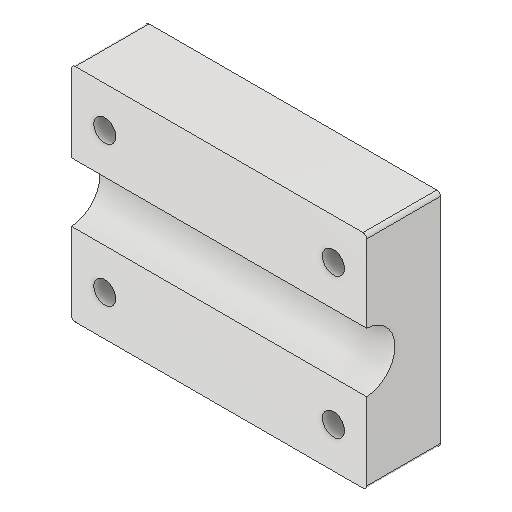
# Autodesk Inventor part: 3DP_PLA_Y_axis_linear_shaft_mount_clamp_with_endstop
Saved by Autodesk Inventor 2025 (Build 290162010, 162A)
## iProperties
Created: 2018-06-17
Part Number: 3DP_PLA_Y_axis_linear_shaft_mount_clamp_with_endstop
Material: ABS Plastic
Document SubType Name: Modeling
Designer: Andrzej
Density: 1.06 g/cm^3
Appearance: Smooth - White
Author: Andrzej
Autodesk Inventor part; units mm, degrees
ref_plane "YZ Plane" through (0, 0, 0) normal (1, 0, 0) x (0, 1, 0)
ref_plane "XZ Plane" through (0, 0, 0) normal (0, 1, 0) x (-1, 0, 0)
ref_plane "XY Plane" through (0, 0, 0) normal (0, 0, 1) x (1, 0, 0)
sketch "Sketch1" plane through (0, 0, 0) normal (0, 0, 1) x (1, 0, 0)
  line L0 (-26.9235, 18.928) -> (13.0765, 18.928)
  line L1 (13.0765, 18.928) -> (13.0765, -11.072)
  line L2 (13.0765, -11.072) -> (-26.9235, -11.072)
  line L3 (-26.9235, -11.072) -> (-26.9235, 18.928)
  point P0 (0, 0)
  dimension "d1" = 30
  dimension "d47" = 40
  constraints: 8 end point, 2 parallel, 1 horizontal, 1 perpendicular
  measures "d1" distance of L0.end L1.end
  measures "d47" distance of L1.end L2.end
extrude "Extrusion1" add sketch "Sketch1" along normal blind 10
sketch "Sketch2" plane through (13.0765, -11.072, 10) normal (1, 0, 0) x (0, 0, -1)
  line L0 (10, 30) -> (0, 30) projected
  line L1 (0, 0) -> (0, 30) projected
  line L2 (10, 0) -> (0, 0) projected
  circle A0 centre (-0.2, 15) radius 4.025
  line L3 (10, 30) -> (10, 0) projected
  dimension "d20" = 30
  dimension "d21" = 15
  dimension "d22" = 0.2
  dimension "d23" = 8.05
  constraints: 1 centre point, 1 coincident
  measures "d20" distance between parallel lines of L0 L2
  measures "d21" distance from line of L2 point (-0.2, 15)
  measures "d22" distance from line of L1 point (-0.2, 15)
  measures "d23" diameter of A0
extrude "Extrusion3" cut sketch "Sketch2" against normal through all contours A0 L1 | L1 A0
sketch "Sketch3" plane through (0, 0, 10) normal (0, 0, 1) x (1, 0, 0)
  line L0 (13.0765, -0.092) -> (-26.9235, -0.092) projected
  line L1 (-26.9235, -0.092) -> (-26.9235, -11.072) projected
  line L2 (-26.9235, -11.072) -> (13.0765, -11.072) projected
  line L3 (13.0765, -11.072) -> (13.0765, -0.092) projected
  line L4 (-26.9235, 7.948) -> (13.0765, 7.948) projected
  line L5 (13.0765, 7.948) -> (13.0765, 18.928) projected
  line L6 (13.0765, 18.928) -> (-26.9235, 18.928) projected
  line L7 (-26.9235, 18.928) -> (-26.9235, 7.948) projected
  point P0 (0, 0)
  point P1 (8.5765, -5.582)
  point P2 (-22.4235, -5.582)
  point P3 (8.5765, 13.438)
  point P4 (-22.4235, 13.438)
  dimension "d26" = 4.5
  dimension "d27" = 10.98
  dimension "d28" = 5.49
  dimension "d29" = 5.49
  dimension "d30" = 4.5
  constraints: 2 horizontal alignment, 2 vertical alignment
  measures "d26" distance from line of L3 point (8.576, -5.582)
  measures "d27" distance between parallel lines of L0 L2
  measures "d28" distance from line of L2 point (8.576, -5.582)
  measures "d29" distance from line of L6 point (8.576, 13.438)
  measures "d30" distance from line of L1 point (-22.424, -5.582)
hole "Hole2" at (8.5765, -5.582, 10) at (-22.4235, -5.582, 10) at (8.5765, 13.438, 10) at (-22.4235, 13.438, 10) direction (0, 0, -1) diameter 3 depth 20 tip angle 118
fillet "Fillet2" radius 0.5 4 edges at (13.0765, 18.928, 5) (-26.9235, 18.928, 5) (13.0765, -11.072, 5) (-26.9235, -11.072, 5)
sketch "Sketch5" plane through (0, 0, 0) normal (0, 0, -1) x (-1, 0, 0)
  arc A0 (26.4235, -11.072) -> (26.9235, -10.572) centre (26.4235, -10.572) ccw projected
  line L0 (26.9235, -10.572) -> (26.9235, 18.428) projected
  arc A1 (26.9235, 18.428) -> (26.4235, 18.928) centre (26.4235, 18.428) ccw projected
  line L1 (26.4235, 18.928) -> (-12.5765, 18.928) projected
  arc A2 (-12.5765, 18.928) -> (-13.0765, 18.428) centre (-12.5765, 18.428) ccw projected
  line L2 (-13.0765, 18.428) -> (-13.0765, -10.572) projected
  arc A3 (-13.0765, -10.572) -> (-12.5765, -11.072) centre (-12.5765, -10.572) ccw projected
  line L3 (-12.5765, -11.072) -> (26.4235, -11.072) projected
  circle A4 centre (-8.5765, 13.438) radius 1.5 projected
  circle A5 centre (-8.5765, -5.582) radius 1.5 projected
  circle A6 centre (22.4235, -5.582) radius 1.5 projected
  circle A7 centre (22.4235, 13.438) radius 1.5 projected
  point P0 (0, 0)
  point P1 (10.9235, -6.822)
  point P2 (10.9235, 14.678)
  dimension "d48" = 4.25
  dimension "d49" = 4.25
  dimension "d50" = 16
  constraints: 1 vertical alignment
  measures "d48" distance from line of L3 point (10.924, -6.822)
  measures "d49" distance from line of L1 point (10.924, 14.678)
  measures "d50" distance from line of L0 point (10.924, -6.822)
hole "Hole4" at (-10.9235, -6.822, 0) at (-10.9235, 14.678, 0) direction (0, 0, 1) diameter 2.5 depth 8 tip angle 118
equation "\"d21\" = 0.5 * d20"
equation "\"d28\" = 0.5 * d27"
equation "\"d29\" = d28"
equation "\"d30\" = d26"
equation "\"d49\" = d48"
body "Solid1"
